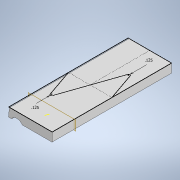
# Autodesk Inventor part: ketchenLightBracketV02
Saved by Autodesk Inventor 2021.2 (Build 252289000, 289)
## iProperties
Created: 2021-01-10
Part Number: ketchenLightBracketV02
Material: Generic
Document SubType Name: Modeling
Designer: robst
Density: 1 g/cm^3
Appearance: Default
Author: robst
Autodesk Inventor part; units mm, degrees
ref_plane "YZ Plane" through (0, 0, 0) normal (1, 0, 0) x (0, 1, 0)
ref_plane "XZ Plane" through (0, 0, 0) normal (0, 1, 0) x (-1, 0, 0)
ref_plane "XY Plane" through (0, 0, 0) normal (0, 0, 1) x (1, 0, 0)
sketch "Sketch2" plane through (0, 0, 0) normal (0, 0, 1) x (1, 0, 0)
  line L0 (0, -33.7271) -> (0, 35.754) construction
  arc A0 (2.8938, 20.8) -> (0, 0) centre (76.2, 0) ccw
  line L1 (101.6, 0) -> (101.6, 20.8)
  line L2 (101.6, 20.8) -> (2.8938, 20.8)
  arc A1 (31.8545, 0) -> (7.0075, 0) centre (19.431, -7.3099) ccw
  line L3 (0, 0) -> (7.0075, 0)
  line L4 (31.8545, 0) -> (101.6, 0)
  dimension "d0" = 152.4
  dimension "d1" = 101.6
  dimension "d2" = 20.8
  dimension "d4" = 28.829
  dimension "d5" = 19.431
  constraints: 10 end point, 4 point on circle, 3 perpendicular, 2 centre point, 2 horizontal, 1 collinear, 1 tangent, 1 vertical
  measures "d0" diameter of A0
  measures "d1" distance of L3.start L1.start
  measures "d2" distance of L1.start L1.end
  measures "d4" diameter of A1
  measures "d5" horizontal distance of A1.centre L3.start
extrude "Extrusion1" add sketch "Sketch2" along normal mid plane 279.4
sketch "Sketch3" plane through (31.8545, 0, 139.7) normal (0, -1, 0) x (1, 0, 0)
  line L0 (69.7455, -279.4) -> (69.7455, 0) construction
  line L1 (0, -279.4) -> (0, 0) construction
  point P0 (-31.8545, -139.7)
  point P1 (58.3155, -12.7)
  dimension "d8" = 11.43
  measures "d8" distance from line of point (58.316, -12.7) L0
hole "Hole2" at (90.17, 0, 127) direction (0, 1, 0) diameter 3.302 depth 15.875 tip angle 118 thread size "8-32 UNC" class "2B" standard "ANSI Unified Screw Threads"
pattern_linear "Rectangular Pattern1" count 8 spacing 6.35 along (-1, 0, 0) of "Hole2"
sketch "SketchForText" plane through (31.8545, 0, 139.7) normal (0, -1, 0) x (1, 0, 0)
  line L0 (69.7455, 0) -> (69.7455, -279.4) construction
  line L1 (69.7455, -139.7) -> (0, -139.7) construction
  line L2 (0, -279.4) -> (0, 0) construction
  line L3 (54.5958, -33.02) -> (57.2202, -25.4)
  line L4 (57.2202, -25.4) -> (58.3132, -25.4)
  line L5 (58.3132, -25.4) -> (60.9376, -33.02)
  line L6 (60.9376, -33.02) -> (59.8508, -33.02)
  line L7 (59.8508, -33.02) -> (57.7389, -26.6906)
  line L8 (57.7389, -26.6906) -> (55.6271, -33.02)
  line L9 (55.6271, -33.02) -> (54.5958, -33.02)
  line L10 (51.2057, -28.2714) -> (54.0895, -28.2714)
  line L11 (54.0895, -28.2714) -> (54.0895, -29.1977)
  line L12 (54.0895, -29.1977) -> (51.2057, -29.1977)
  line L13 (51.2057, -29.1977) -> (51.2057, -28.2714)
  spline S0 degree 2 poles (45.4506, -29.21) (45.4506, -27.1599) (46.6424, -25.2394) (47.8836, -25.2394) knots 0 0 0 1 2 2 2
  spline S1 degree 2 poles (47.8836, -25.2394) (49.1433, -25.2394) (50.3227, -27.1969) (50.3227, -29.2038) knots 0 0 0 1 2 2 2
  spline S2 degree 2 poles (50.3227, -29.2038) (50.3227, -31.2663) (49.1309, -33.1744) (47.8836, -33.1744) knots 0 0 0 1 2 2 2
  spline S3 degree 2 poles (47.8836, -33.1744) (46.63, -33.1744) (45.4506, -31.1984) (45.4506, -29.21) knots 0 0 0 1 2 2 2
  spline S4 degree 2 poles (46.7597, -26.8882) (46.6115, -27.2649) (46.488, -28.4258) (46.488, -29.21) knots 0 0 0 1 2 2 2
  spline S5 degree 2 poles (46.488, -29.21) (46.488, -29.9942) (46.6115, -31.149) (46.7659, -31.538) knots 0 0 0 1 2 2 2
  spline S6 degree 2 poles (46.7659, -31.538) (46.9203, -31.927) (47.4575, -32.3284) (47.8836, -32.3284) knots 0 0 0 1 2 2 2
  spline S7 degree 2 poles (47.8836, -32.3284) (48.3096, -32.3284) (48.8592, -31.927) (49.0198, -31.5256) knots 0 0 0 1 2 2 2
  spline S8 degree 2 poles (49.0198, -31.5256) (49.1741, -31.1366) (49.2853, -29.951) (49.2853, -29.2038) knots 0 0 0 1 2 2 2
  spline S9 degree 2 poles (49.2853, -29.2038) (49.2853, -28.4011) (49.1865, -27.3266) (49.0259, -26.9067) knots 0 0 0 1 2 2 2
  spline S10 degree 2 poles (49.0259, -26.9067) (48.8777, -26.5115) (48.3282, -26.0854) (47.8836, -26.0854) knots 0 0 0 1 2 2 2
  spline S11 degree 2 poles (47.8836, -26.0854) (47.4637, -26.0854) (46.9141, -26.4868) (46.7597, -26.8882) knots 0 0 0 1 2 2 2
  line L14 (39.7757, -25.4) -> (44.4749, -25.4)
  line L15 (44.4749, -25.4) -> (44.4749, -26.4806)
  spline S12 degree 2 poles (44.4749, -26.4806) (43.9686, -26.9561) (43.067, -27.8391) (42.6348, -28.3146) knots 0 0 0 1 2 2 2
  spline S13 degree 2 poles (42.6348, -28.3146) (41.7641, -29.2718) (41.1281, -30.4203) (41.1281, -31.0316) knots 0 0 0 1 2 2 2
  spline S14 degree 2 poles (41.1281, -31.0316) (41.1281, -31.3527) (41.3257, -31.8344) (41.5047, -31.9888) knots 0 0 0 1 2 2 2
  spline S15 degree 2 poles (41.5047, -31.9888) (41.6838, -32.1431) (42.1531, -32.2975) (42.4372, -32.2975) knots 0 0 0 1 2 2 2
  spline S16 degree 2 poles (42.4372, -32.2975) (42.7089, -32.2975) (43.2646, -32.1617) (43.5178, -32.0567) knots 0 0 0 1 2 2 2
  spline S17 degree 2 poles (43.5178, -32.0567) (43.7339, -31.9702) (44.1353, -31.7232) (44.2588, -31.6368) knots 0 0 0 1 2 2 2
  line L16 (44.2588, -31.6368) -> (44.3144, -31.6368)
  line L17 (44.3144, -31.6368) -> (44.3144, -32.7236)
  spline S18 degree 2 poles (44.3144, -32.7236) (43.9995, -32.878) (42.8694, -33.1806) (42.3631, -33.1806) knots 0 0 0 1 2 2 2
  spline S19 degree 2 poles (42.3631, -33.1806) (41.2948, -33.1806) (40.0907, -32.0505) (40.0907, -31.0872) knots 0 0 0 1 2 2 2
  spline S20 degree 2 poles (40.0907, -31.0872) (40.0907, -30.6364) (40.3006, -29.8831) (40.4859, -29.562) knots 0 0 0 1 2 2 2
  spline S21 degree 2 poles (40.4859, -29.562) (40.6711, -29.2285) (41.2083, -28.574) (41.5047, -28.259) knots 0 0 0 1 2 2 2
  spline S22 degree 2 poles (41.5047, -28.259) (41.9864, -27.7342) (43.1658, -26.6103) (43.5178, -26.283) knots 0 0 0 1 2 2 2
  line L18 (43.5178, -26.283) -> (39.7757, -26.283)
  line L19 (39.7757, -26.283) -> (39.7757, -25.4)
  spline S23 degree 2 poles (30.4514, -30.7229) (30.4514, -30.2289) (30.8034, -29.3397) (31.1183, -29.0309) knots 0 0 0 1 2 2 2
  spline S24 degree 2 poles (31.1183, -29.0309) (31.5135, -28.6419) (32.5818, -28.2405) (33.3969, -28.2405) knots 0 0 0 1 2 2 2
  line L20 (33.3969, -28.2405) -> (34.2552, -28.2405)
  line L21 (34.2552, -28.2405) -> (34.2552, -25.4)
  line L22 (34.2552, -25.4) -> (35.268, -25.4)
  line L23 (35.268, -25.4) -> (35.268, -33.02)
  line L24 (35.268, -33.02) -> (33.3537, -33.02)
  spline S25 degree 2 poles (33.3537, -33.02) (32.6744, -33.02) (31.7235, -32.7977) (31.3592, -32.5445) knots 0 0 0 1 2 2 2
  spline S26 degree 2 poles (31.3592, -32.5445) (30.9331, -32.2543) (30.4514, -31.3589) (30.4514, -30.7229) knots 0 0 0 1 2 2 2
  spline S27 degree 2 poles (31.5074, -30.692) (31.5074, -31.0872) (31.7791, -31.6677) (32.0569, -31.8529) knots 0 0 0 1 2 2 2
  spline S28 degree 2 poles (32.0569, -31.8529) (32.2978, -32.0135) (32.94, -32.1431) (33.4154, -32.1431) knots 0 0 0 1 2 2 2
  line L25 (33.4154, -32.1431) -> (34.2552, -32.1431)
  line L26 (34.2552, -32.1431) -> (34.2552, -29.105)
  line L27 (34.2552, -29.105) -> (33.5636, -29.105)
  spline S29 degree 2 poles (33.5636, -29.105) (32.9461, -29.105) (32.1866, -29.3026) (31.9396, -29.562) knots 0 0 0 1 2 2 2
  spline S30 degree 2 poles (31.9396, -29.562) (31.7111, -29.7905) (31.5074, -30.3277) (31.5074, -30.692) knots 0 0 0 1 2 2 2
  line L28 (23.9615, -33.02) -> (26.5858, -25.4)
  line L29 (26.5858, -25.4) -> (27.6788, -25.4)
  line L30 (27.6788, -25.4) -> (30.3032, -33.02)
  line L31 (30.3032, -33.02) -> (29.2164, -33.02)
  line L32 (29.2164, -33.02) -> (27.1045, -26.6906)
  line L33 (27.1045, -26.6906) -> (24.9927, -33.02)
  line L34 (24.9927, -33.02) -> (23.9615, -33.02)
  line L35 (20.5714, -28.2714) -> (23.4551, -28.2714)
  line L36 (23.4551, -28.2714) -> (23.4551, -29.1977)
  line L37 (23.4551, -29.1977) -> (20.5714, -29.1977)
  line L38 (20.5714, -29.1977) -> (20.5714, -28.2714)
  spline S31 degree 2 poles (14.8162, -29.21) (14.8162, -27.1599) (16.008, -25.2394) (17.2492, -25.2394) knots 0 0 0 1 2 2 2
  spline S32 degree 2 poles (17.2492, -25.2394) (18.5089, -25.2394) (19.6883, -27.1969) (19.6883, -29.2038) knots 0 0 0 1 2 2 2
  spline S33 degree 2 poles (19.6883, -29.2038) (19.6883, -31.2663) (18.4965, -33.1744) (17.2492, -33.1744) knots 0 0 0 1 2 2 2
  spline S34 degree 2 poles (17.2492, -33.1744) (15.9957, -33.1744) (14.8162, -31.1984) (14.8162, -29.21) knots 0 0 0 1 2 2 2
  spline S35 degree 2 poles (16.1253, -26.8882) (15.9771, -27.2649) (15.8536, -28.4258) (15.8536, -29.21) knots 0 0 0 1 2 2 2
  spline S36 degree 2 poles (15.8536, -29.21) (15.8536, -29.9942) (15.9771, -31.149) (16.1315, -31.538) knots 0 0 0 1 2 2 2
  spline S37 degree 2 poles (16.1315, -31.538) (16.2859, -31.927) (16.8231, -32.3284) (17.2492, -32.3284) knots 0 0 0 1 2 2 2
  spline S38 degree 2 poles (17.2492, -32.3284) (17.6753, -32.3284) (18.2248, -31.927) (18.3854, -31.5256) knots 0 0 0 1 2 2 2
  spline S39 degree 2 poles (18.3854, -31.5256) (18.5398, -31.1366) (18.6509, -29.951) (18.6509, -29.2038) knots 0 0 0 1 2 2 2
  spline S40 degree 2 poles (18.6509, -29.2038) (18.6509, -28.4011) (18.5521, -27.3266) (18.3916, -26.9067) knots 0 0 0 1 2 2 2
  spline S41 degree 2 poles (18.3916, -26.9067) (18.2434, -26.5115) (17.6938, -26.0854) (17.2492, -26.0854) knots 0 0 0 1 2 2 2
  spline S42 degree 2 poles (17.2492, -26.0854) (16.8293, -26.0854) (16.2797, -26.4868) (16.1253, -26.8882) knots 0 0 0 1 2 2 2
  spline S43 degree 2 poles (9.024, -27.87) (9.024, -27.2834) (9.4131, -26.2892) (9.7403, -25.9558) knots 0 0 0 1 2 2 2
  spline S44 degree 2 poles (9.7403, -25.9558) (10.08, -25.6038) (10.9321, -25.2394) (11.4446, -25.2394) knots 0 0 0 1 2 2 2
  spline S45 degree 2 poles (11.4446, -25.2394) (11.9572, -25.2394) (12.8032, -25.5853) (13.1243, -25.9311) knots 0 0 0 1 2 2 2
  spline S46 degree 2 poles (13.1243, -25.9311) (13.5195, -26.3448) (13.9641, -27.7342) (13.9641, -28.7469) knots 0 0 0 1 2 2 2
  spline S47 degree 2 poles (13.9641, -28.7469) (13.9641, -29.7411) (13.5565, -31.3404) (13.1304, -31.9332) knots 0 0 0 1 2 2 2
  spline S48 degree 2 poles (13.1304, -31.9332) (12.7167, -32.5136) (11.4076, -33.162) (10.5493, -33.162) knots 0 0 0 1 2 2 2
  spline S49 degree 2 poles (10.5493, -33.162) (10.2961, -33.162) (9.8515, -33.1126) (9.6848, -33.0571) knots 0 0 0 1 2 2 2
  line L39 (9.6848, -33.0571) -> (9.6848, -32.0752)
  line L40 (9.6848, -32.0752) -> (9.728, -32.0752)
  spline S50 degree 2 poles (9.728, -32.0752) (9.87, -32.1493) (10.3887, -32.279) (10.6851, -32.279) knots 0 0 0 1 2 2 2
  spline S51 degree 2 poles (10.6851, -32.279) (11.6361, -32.279) (12.8032, -30.9946) (12.9143, -29.7349) knots 0 0 0 1 2 2 2
  spline S52 degree 2 poles (12.9143, -29.7349) (12.55, -29.9881) (11.7843, -30.2659) (11.3273, -30.2659) knots 0 0 0 1 2 2 2
  spline S53 degree 2 poles (11.3273, -30.2659) (10.8827, -30.2659) (10.2158, -30.0869) (9.8515, -29.8152) knots 0 0 0 1 2 2 2
  spline S54 degree 2 poles (9.8515, -29.8152) (9.4316, -29.5002) (9.024, -28.5246) (9.024, -27.87) knots 0 0 0 1 2 2 2
  spline S55 degree 2 poles (10.0614, -27.8268) (10.0614, -28.2961) (10.3084, -28.9321) (10.5801, -29.1544) knots 0 0 0 1 2 2 2
  spline S56 degree 2 poles (10.5801, -29.1544) (10.7839, -29.315) (11.2903, -29.42) (11.5558, -29.42) knots 0 0 0 1 2 2 2
  spline S57 degree 2 poles (11.5558, -29.42) (11.9139, -29.42) (12.587, -29.2038) (12.9143, -29) knots 0 0 0 1 2 2 2
  spline S58 degree 2 poles (12.9143, -29) (12.9205, -28.8889) (12.9328, -28.6789) (12.9328, -28.5184) knots 0 0 0 1 2 2 2
  spline S59 degree 2 poles (12.9328, -28.5184) (12.9328, -27.728) (12.6241, -26.7585) (12.3894, -26.5053) knots 0 0 0 1 2 2 2
  spline S60 degree 2 poles (12.3894, -26.5053) (12.1733, -26.2645) (11.704, -26.0731) (11.4385, -26.0731) knots 0 0 0 1 2 2 2
  spline S61 degree 2 poles (11.4385, -26.0731) (10.821, -26.0731) (10.0614, -26.9499) (10.0614, -27.8268) knots 0 0 0 1 2 2 2
  point P0 (-31.8545, -139.7)
  constraints: 2 end point, 2 midpoint, 1 horizontal
extrude "ExtrusionForText" cut sketch "SketchForText" against normal blind 1.27
sketch "SketchForSplittingPart" plane through (2.8938, 20.8, 139.7) normal (0, 1, 0) x (1, 0, 0)
  line L0 (-2.8938, 279.4) -> (-2.8938, 0) projected
  line L1 (0, 279.4) -> (98.7062, 279.4) projected
  line L2 (98.7062, 279.4) -> (98.7062, 0) projected
  line L3 (98.7062, 0) -> (0, 0) projected
  line L4 (-2.8938, 0) -> (98.7062, 0)
  line L5 (98.7062, 0) -> (98.7062, 279.4)
  line L6 (98.7062, 279.4) -> (-2.8938, 279.4)
  line L7 (-2.8938, 279.4) -> (-2.8938, 0)
  line L8 (98.7062, 139.7) -> (-2.8938, 139.7) construction
  line L9 (47.9062, 139.7) -> (47.9062, 279.4) construction
  line L10 (98.7062, 139.7) -> (76.3082, 204.7334)
  line L11 (70.3043, 204.7334) -> (47.9062, 139.7)
  line L12 (47.9062, 139.7) -> (25.5082, 74.6666)
  line L13 (56.6395, 25.4) -> (59.2639, 33.02) projected
  line L14 (19.5043, 74.6666) -> (-2.8938, 139.7)
  arc A0 (76.3082, 204.7334) -> (70.3043, 204.7334) centre (73.3062, 203.6995) ccw
  arc A1 (19.5043, 74.6666) -> (25.5082, 74.6666) centre (22.5062, 75.7005) ccw
  dimension "d30" = 3.175
  dimension "d31" = 3.175
  constraints: 20 end point, 4 parallel, 4 point on circle, 4 tangent, 3 equal length, 3 midpoint, 2 centre point, 2 perpendicular, 1 horizontal, 1 point on line
  measures "d30" radius of A0
  measures "d31" radius of A1
ref_plane "Work Plane1" through (0, 0, 88.9) normal (0, 0, 1) x (1, 0, 0)
equation "\"d0\" = 2 * radiusOfCurvatureForWall"
equation "\"d1\" = distanceFromWall"
equation "\"d2\" = thickness"
equation "\"d4\" = dometicDiameter"
equation "\"d5\" = dometicCenterDistanceFromWall"
equation "\"d6\" = width"
equation "\"d8\" = startingHole"
equation "\"thickness\" = 20.8"
equation "\"distanceFromWall\" = 101.6"
equation "\"radiusOfCurvatureForWall\" = 76.2"
equation "\"dometicDiameter\" = 28.829"
equation "\"dometicCenterDistanceFromWall\" = 19.431"
equation "\"startingHole\" = 11.43"
equation "\"width\" = 279.4"
body "Solid1"
